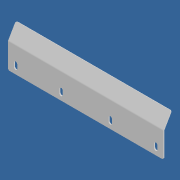
# Autodesk Inventor part: Scraper_Bar
Saved by Autodesk Inventor 2020 (Build 240168000, 168)
## iProperties
Created: 2021-05-29
Part Number: Scraper_Bar
Material: 一般
Document SubType Name: Sheet Metal
Designer: ken113
Density: 1 g/cm^3
Sheet Metal Rule: Default_mm
Appearance: 既定
Flat Pattern Width: 5.33271 cm
Flat Pattern Length: 20.5 cm
Flat Pattern Area: 109.321 cm^2
Sheet Metal Width: 53.327 mm
Sheet Metal Length: 205.000 mm
Sheet Metal Area: 10932.061 mm^2
Author: ken113
Autodesk Inventor part; units mm, degrees
ref_plane "YZ Plane" through (0, 0, 0) normal (1, 0, 0) x (0, 1, 0)
ref_plane "XZ Plane" through (0, 0, 0) normal (0, 1, 0) x (-1, 0, 0)
ref_plane "XY Plane" through (0, 0, 0) normal (0, 0, 1) x (1, 0, 0)
sketch "スケッチ1" plane through (0, 0, 0) normal (0, 0, 1) x (1, 0, 0)
  line L0 (102.5, -16.5) -> (-102.5, -16.5)
  line L1 (-102.5, -16.5) -> (-102.5, 16.5)
  line L2 (-102.5, 16.5) -> (102.5, 16.5)
  line L3 (102.5, 16.5) -> (102.5, -16.5)
  line L4 (102.5, -16.5) -> (-102.5, 16.5) construction
  line L5 (-102.5, -16.5) -> (102.5, 16.5) construction
  point P0 (0, 0)
  dimension "d0" = 205
  dimension "d1" = 33
  measures "d0" distance of L1.end L2.end
  measures "d1" distance of L0.end L1.end
extrude "プレート1" add sketch "スケッチ1" along normal blind 1.5
sketch "スケッチ2" plane through (102.5, 16.5, 0) normal (0, 0.5, 0.8660254) x (-1, 0, 0)
  line L0 (205, 0) -> (0, 0)
  line L1 (0, 0) -> (0, -20)
  line L2 (0, -20) -> (205, -20)
  line L3 (205, -20) -> (205, 0)
  constraints: 6 end point, 1 horizontal, 1 perpendicular, 1 vertical
edge flange "フランジ1" height 20 angle 30 thickness 1.5 bend radius 1.5 thickness toward (0, 0.5, 0.8660254) relief tear relief width 1.5 relief depth 0.75 edges at (0, 16.5, 0) wall of the first edge with corners at (-102.5, 16.5, 0) (102.5, 16.5, 0) (102.5, 33.8205, -10) (-102.5, 33.8205, -10)
bend "曲げ1"
corner "コーナー1"
sketch "スケッチ3" plane through (0, 0, 1.5) normal (0, 0, 1) x (1, 0, 0)
  line L0 (102.5, 16.0981) -> (-102.5, 16.0981) projected
  line L1 (-102.5, -16.5) -> (-102.5, 16.0981) projected
  line L2 (102.5, -16.5) -> (-102.5, -16.5) projected
  line L3 (102.5, 16.0981) -> (102.5, -16.5) projected
  point P0 (0, 0)
  point P1 (-92.5, -6.5)
  point P2 (92.5, -6.5)
  point P3 (-32.5, -6.5)
  point P4 (32.5, -6.5)
  dimension "d13" = 10
  dimension "d14" = 10
  dimension "d15" = 10
  dimension "d16" = 185
  dimension "d32" = 60
  dimension "d33" = 60
  constraints: 1 horizontal alignment
  measures "d13" distance from line of point (92.5, -6.5) L2
  measures "d14" distance from line of point (-92.5, -6.5) L1
  measures "d15" distance from line of L3 point (92.5, -6.5)
  measures "d16" distance of point (92.5, -6.5) point (-92.5, -6.5)
  measures "d32" distance of point (-32.5, -6.5) point (-92.5, -6.5)
  measures "d33" distance of point (92.5, -6.5) point (32.5, -6.5)
hole "穴1" at (-92.5, -6.5, 1.5) at (92.5, -6.5, 1.5) at (-32.5, -6.5, 1.5) at (32.5, -6.5, 1.5) direction (0, 0, -1) diameter 4.5 end through all
fillet "フィレット1" radius 2 4 edges at (-102.5, -16.5, 0.75) (-102.5, 34.1955, -9.3505) (102.5, 34.1955, -9.3505) (102.5, -16.5, 0.75)
sketch "スケッチ4" plane through (0, 0, 1.5) normal (0, 0, 1) x (1, 0, 0)
  circle A0 centre (-32.5, -6.5) radius 2.25 projected
  circle A1 centre (-92.5, -6.5) radius 2.25 projected
  circle A2 centre (92.5, -6.5) radius 2.25 projected
  circle A3 centre (32.5, -6.5) radius 2.25 projected
  arc A4 (100.5, -16.5) -> (102.5, -14.5) centre (100.5, -14.5) ccw projected
  line L0 (102.5, 16.0981) -> (102.5, -14.5) projected
  line L1 (102.5, 16.0981) -> (-102.5, 16.0981) projected
  line L2 (-102.5, -14.5) -> (-102.5, 16.0981) projected
  arc A5 (-102.5, -14.5) -> (-100.5, -16.5) centre (-100.5, -14.5) ccw projected
  line L3 (100.5, -16.5) -> (-100.5, -16.5) projected
  line L4 (-92.5, -4) -> (-92.5, -9) construction
  line L5 (-94.75, -4) -> (-94.75, -9)
  line L6 (-90.25, -9) -> (-90.25, -4)
  arc A6 (-90.25, -4) -> (-94.75, -4) centre (-92.5, -4) ccw
  arc A7 (-94.75, -9) -> (-90.25, -9) centre (-92.5, -9) ccw
  line L7 (-32.5, -9) -> (-32.5, -4) construction
  line L8 (-30.25, -9) -> (-30.25, -4)
  line L9 (-34.75, -4) -> (-34.75, -9)
  arc A8 (-34.75, -9) -> (-30.25, -9) centre (-32.5, -9) ccw
  arc A9 (-30.25, -4) -> (-34.75, -4) centre (-32.5, -4) ccw
  line L10 (32.5, -9) -> (32.5, -4) construction
  circle A10 centre (32.5, -6.5) radius 2.25 projected
  line L11 (30.25, -9) -> (30.25, -4)
  line L12 (34.75, -4) -> (34.75, -9)
  arc A11 (30.25, -9) -> (34.75, -9) centre (32.5, -9) ccw
  arc A12 (34.75, -4) -> (30.25, -4) centre (32.5, -4) ccw
  line L13 (92.5, -9) -> (92.5, -4) construction
  line L14 (90.25, -9) -> (90.25, -4)
  line L15 (94.75, -4) -> (94.75, -9)
  arc A13 (90.25, -9) -> (94.75, -9) centre (92.5, -9) ccw
  arc A14 (94.75, -4) -> (90.25, -4) centre (92.5, -4) ccw
  circle A15 centre (-32.5, -6.5) radius 2.25 projected
  circle A16 centre (-92.5, -6.5) radius 2.25 projected
  point P0 (0, 0)
  dimension "d34" = 5
  constraints: 32 end point, 20 tangent, 16 point on circle, 8 centre point, 6 parallel, 4 midpoint, 3 horizontal alignment, 2 vertical
  measures "d34" distance of L4.start L4.end
extrude "押し出し1" cut sketch "スケッチ4" against normal blind 10 contours A0 | L8 A8 L9 A0 | A0 L9 A9 L8 | A1 | L6 A7 L5 A1 | A1 L5 A6 L6 | A2 | L15 A13 L14 A2 | A2 L14 A14 L15 | A3 | L12 A11 L11 A3 | A3 L11 A12 L12
equation "\"d29\" = Thickness"
equation "\"d2\" = Thickness"
equation "\"d3\" = BendReliefWidth"
equation "\"d4\" = BendReliefDepth"
equation "\"d5\" = MinimumRemnant"
equation "\"d6\" = TransitionRadius"
equation "\"d9\" = BendRadius"
equation "\"d10\" = CornerReliefSize"
equation "\"d11\" = GapSize"
equation "\"d12\" = JacobiRadiusSize"
equation "\"BendRadius\" = Thickness"
equation "\"BendReliefWidth\" = Thickness"
equation "\"BendReliefDepth\" = 0.5 * Thickness"
equation "\"CornerReliefSize\" = 4 * Thickness"
equation "\"MinimumRemnant\" = 2 * Thickness"
equation "\"TransitionRadius\" = BendRadius"
equation "\"JacobiRadiusSize\" = BendRadius"
equation "\"GapSize\" = Thickness"
equation "\"Thickness\" = 1.5"
